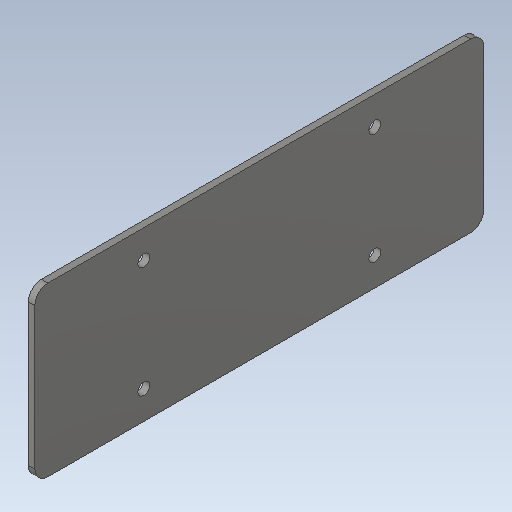
# Autodesk Inventor part: ZaslepkaObudowa
Saved by Autodesk Inventor 2020 (Build 240168000, 168)
## iProperties
Created: 2020-08-21
Part Number: ZaslepkaObudowa
Material: Aluminum 6061
Document SubType Name: Konstrukcja blachowa
Designer: barto
Density: 2.7 g/cm^3
Sheet Metal Rule: Default_mm
Appearance: Aluminum - Flat
Flat Pattern Width: 7.7 cm
Flat Pattern Length: 20.6 cm
Flat Pattern Area: 158.62 cm^2
Sheet Metal Width: 77,000 mm
Sheet Metal Length: 206,000 mm
Sheet Metal Area: 15862,000 mm^2
Author: barto
Autodesk Inventor part; units mm, degrees
ref_plane "YZ Plane" through (0, 0, 0) normal (1, 0, 0) x (0, 1, 0)
ref_plane "XZ Plane" through (0, 0, 0) normal (0, 1, 0) x (-1, 0, 0)
ref_plane "XY Plane" through (0, 0, 0) normal (0, 0, 1) x (1, 0, 0)
sketch "Szkic1" plane through (0, 0, 0) normal (1, 0, 0) x (0, 1, 0)
  line L0 (-32.5, 103) -> (32.5, 103)
  line L1 (38.5, 97) -> (38.5, -97)
  line L2 (32.5, -103) -> (-32.5, -103)
  line L3 (-38.5, -97) -> (-38.5, 97)
  line L4 (-38.5, 103) -> (38.5, -103) construction
  arc A0 (32.5, -103) -> (38.5, -97) centre (32.5, -97) ccw
  arc A1 (-32.5, 103) -> (-38.5, 97) centre (-32.5, 97) ccw
  arc A2 (-38.5, -97) -> (-32.5, -103) centre (-32.5, -97) ccw
  arc A3 (38.5, 97) -> (32.5, 103) centre (32.5, 97) ccw
  point P0 (0, 0)
  dimension "d3" = 6
  measures "d3" radius of A0
extrude "Płyta1" add sketch "Szkic1" along normal blind 3
sketch "Szkic2" plane through (3, 0, 0) normal (1, 0, 0) x (0, 0, -1)
  line L0 (-97, 38.5) -> (97, 38.5) projected
  line L1 (-103, -32.5) -> (-103, 32.5) projected
  line L2 (103, 32.5) -> (103, -32.5) projected
  line L3 (97, -38.5) -> (-97, -38.5) projected
  point P0 (0, 0)
  point P1 (-53, 25.5)
  point P2 (53, 25.5)
  point P3 (53, -25.5)
  point P4 (-53, -25.5)
  dimension "d5" = 13
  dimension "d6" = 50
  dimension "d7" = 50
  dimension "d8" = 13
  dimension "d9" = 50
  dimension "d10" = 13
  dimension "d11" = 13
  dimension "d12" = 50
  measures "d5" distance from line of L0 point (-53, 25.5)
  measures "d6" distance from line of L1 point (-53, 25.5)
  measures "d7" distance from line of L2 point (53, 25.5)
  measures "d8" distance from line of L0 point (53, 25.5)
  measures "d9" distance from line of L2 point (53, -25.5)
  measures "d10" distance from line of L3 point (53, -25.5)
  measures "d11" distance from line of L3 point (-53, -25.5)
  measures "d12" distance from line of L1 point (-53, -25.5)
hole "Otwór1" at (3, -25.5, 53) at (3, 25.5, 53) at (3, 25.5, -53) at (3, -25.5, -53) direction (-1, 0, 0) diameter 5.5 depth 3 tip angle 118 clearance for "Śruba ze łbem płaskim obrobiona" size "M5" standard "ANSI Profil metryczny M"
equation "\"d18\" = Grubość"
equation "\"d4\" = Grubość"
equation "\"PromieńGięcia\" = Grubość"
equation "\"SzerokośćGięciaPodcięcia\" = Grubość"
equation "\"GłębokośćGięciaPodcięcia\" = 0.5 * Grubość"
equation "\"RozmiarPodcięciaNarożnika\" = 4 * Grubość"
equation "\"MinimalnaPozostałość\" = 2 * Grubość"
equation "\"PromieńPrzejścia\" = PromieńGięcia"
equation "\"Rozmiar_promienia_Jacobiego\" = PromieńGięcia"
equation "\"Wielk_odstępu\" = Grubość"
equation "\"Grubość\" = 3"
